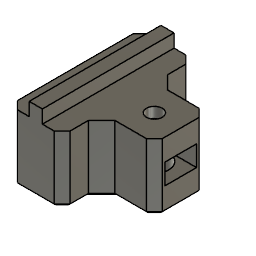
triple leg for power supply (Autodesk Fusion 360 design; units mm, degrees)
Autodesk Fusion 360 part; units mm, degrees
sketch "Szkic1" plane through (0, 0, 0) normal (0, 0, 1) x (1, 0, 0)
  line L0 (-20, 25) -> (-20, -25)
  line L1 (-20, -25) -> (0, -25)
  line L2 (0, -25) -> (0, 25)
  line L3 (0, 25) -> (-20, 25)
  line L4 (0, 10) -> (0, -10)
  line L5 (0, -10) -> (20, -10)
  line L6 (20, -10) -> (20, 10)
  line L7 (20, 10) -> (0, 10)
  circle A0 centre (10, 0) radius 3
  circle A1 centre (10, 0) radius 5.5
  line L8 (-12.5, 25) -> (-7.5, 25)
  line L9 (-7.5, 25) -> (-7.5, -25)
  line L10 (-7.5, -25) -> (-12.5, -25)
  line L11 (-12.5, -25) -> (-12.5, 25)
  dimension "d1" = 6
  dimension "d2" = 11
  constraint perpendicular L0 L1
  constraint parallel L0 L2
  constraint parallel L1 L3
  constraint vertical L0
  constraint perpendicular L4 L5
  constraint parallel L4 L6
  constraint parallel L5 L7
  constraint coincident L2 L4.end
  constraint parallel L2 L4
  constraint concentric A0 A1
  constraint perpendicular L8 L9
  constraint parallel L8 L10
  constraint parallel L9 L11
  constraint coincident L3 L8.end
  constraint coincident L3 L8.start
  measures "d1" diameter of A0
  measures "d2" diameter of A1
extrude "Wyciągnięcie proste1" add sketch "Szkic1" against normal blind 25 contours L0 L1 L3 L11 | L1 L3 L8 L9 L10 L11 | L1 L2 L3 L4 L9 | L2 L4 L5 L6 L7
extrude "Wyciągnięcie proste2" add sketch "Szkic1" against normal blind 4.2 contours A0 | A1
extrude "Wyciągnięcie proste3" cut sketch "Szkic1" against normal blind 4 contours A0
extrude "Wyciągnięcie proste4" add sketch "Szkic1" along normal blind 5 contours L1 L3 L8 L9 L10 L11
chamfer "Fazowanie1" distance 5 angle 45 1 edges at (0, -10, -12.5)
chamfer "Fazowanie2" distance 5 angle 45 1 edges at (0, 10, -12.5)
chamfer "Fazowanie3" distance 3 angle 45 6 edges at (20, 10, -12.5) (20, -10, -12.5) (0, 25, -12.5) (-20, 25, -12.5) (-20, -25, -12.5) (0, -25, -12.5)
chamfer "Fazowanie4" distance 1 angle 45 1 faces at (-11.8333, 0, -25)
delete_face "Usuń powierzchnię1" 1 faces at (16.159, -0.3074, -24.6667)
sketch "Szkic2" plane through (-20, 0, 0) normal (-1, 0, 0) x (0, -1, 0)
  line L0 (-22, -24) -> (22, -24)
  line L1 (22, -24) -> (22, 0)
  line L2 (22, 0) -> (-22, 0)
  line L3 (-22, 0) -> (-22, -24)
  line L4 (0, -12) -> (12.5, -12)
  line L5 (0, -12) -> (-12.5, -12)
  line L6 (0, -12) -> (12.5, -12)
  line L7 (0, -12) -> (-12.5, -12)
  line L8 (17.5, -4.5) -> (-17.5, -4.5)
  line L9 (-17.5, -4.5) -> (-17.5, -19.5)
  line L10 (-17.5, -19.5) -> (17.5, -19.5)
  line L11 (17.5, -19.5) -> (17.5, -4.5)
  line L12 (17.5, -4.5) -> (-17.5, -19.5) construction
  line L13 (-17.5, -4.5) -> (17.5, -19.5) construction
  line L14 (11, -5.5) -> (-11, -5.5)
  line L15 (-11, -5.5) -> (-11, -18.5)
  line L16 (-11, -18.5) -> (11, -18.5)
  line L17 (11, -18.5) -> (11, -5.5)
  line L18 (11, -5.5) -> (-11, -18.5) construction
  line L19 (-11, -5.5) -> (11, -18.5) construction
  circle A0 centre (-14.25, -12) radius 2
  circle A1 centre (14.25, -12) radius 2
  line L20 (6, -16) -> (-6, -16)
  line L21 (-6, -16) -> (-6, -8)
  line L22 (-6, -8) -> (6, -8)
  line L23 (6, -8) -> (6, -16)
  line L24 (6, -16) -> (-6, -8) construction
  line L25 (-6, -16) -> (6, -8) construction
  point P0 (0, -12)
  point P1 (0, -12)
  point P2 (0, -12)
  dimension "d15" = 12.5
  dimension "d16" = 12.5
  dimension "d18" = 4
  dimension "d19" = 4
  constraint horizontal L4
  constraint parallel L4 L5
  constraint parallel L4 L6
  constraint parallel L5 L7
  constraint horizontal L8
  constraint perpendicular L8 L9
  constraint parallel L8 L10
  constraint parallel L9 L11
  constraint coincident L12 P2
  constraint coincident L13 P2
  constraint coincident P2 P1
  constraint horizontal L14
  constraint perpendicular L14 L15
  constraint parallel L14 L16
  constraint parallel L15 L17
  constraint coincident L18 P2
  constraint coincident L19 P2
  constraint horizontal L20
  constraint perpendicular L20 L21
  constraint parallel L20 L22
  constraint parallel L21 L23
  constraint coincident L24 P2
  constraint coincident L25 P2
  measures "d15" distance of P2 L4.end
  measures "d16" distance of P2 L5.end
  measures "d18" diameter of A0
  measures "d19" diameter of A1
extrude "Wyciągnięcie proste5" cut sketch "Szkic2" against normal blind 15 contours L4 L5 L6 L7 L21 L22 L23 | L4 L5 L6 L7 L20 L21 L23 | L4 L5 L6 L7 L14 L15 L17 L21 L22 L23 | L4 L5 L6 L7 L15 L16 L17 L20 L21 L23
extrude "Wyciągnięcie proste6" cut sketch "Szkic2" against normal blind 300 contours L4 L5 L6 L7 L21 L22 L23 | L4 L5 L6 L7 L20 L21 L23
extrude "Wyciągnięcie proste7" cut sketch "Szkic2" against normal blind 15 contours A0 | A1
sketch "Szkic3" plane through (0, 0, -8) normal (0, 0, -1) x (1, 0, 0)
  line L0 (-5, 6) -> (-5, -6)
  line L1 (-5, -6) -> (20, -6)
  line L2 (20, -6) -> (20, 6)
  line L3 (20, 6) -> (-5, 6)
  circle A0 centre (10, 0) radius 5.5
extrude "Wyciągnięcie proste8" add sketch "Szkic3" along normal blind 0.2 contours L0 L1 L2 L3 | A0
